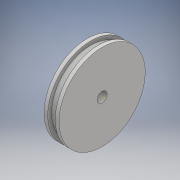
# Autodesk Inventor part: Roue_encodeuse
Saved by Autodesk Inventor 2018 (Build 220112000, 112)
## iProperties
Created: 2019-11-11
Part Number: Roue_encodeuse
Material: Generic
Document SubType Name: Modeling
Designer: hugo
Density: 1 g/cm^3
Appearance: Default
Author: hugo
Autodesk Inventor part; units mm, degrees
ref_plane "YZ Plane" through (0, 0, 0) normal (1, 0, 0) x (0, 1, 0)
ref_plane "XZ Plane" through (0, 0, 0) normal (0, 1, 0) x (-1, 0, 0)
ref_plane "XY Plane" through (0, 0, 0) normal (0, 0, 1) x (1, 0, 0)
sketch "Sketch4" plane through (0, 0, 0) normal (0, 1, 0) x (-1, 0, 0)
  line L0 (0, 0) -> (0, 17.25)
  line L1 (0, 17.25) -> (1.5, 17.25)
  line L2 (1.5, 17.25) -> (1.5, 15.75)
  line L3 (1.5, 15.75) -> (4.5, 15.75)
  line L4 (4.5, 15.75) -> (4.5, 17.25)
  line L5 (4.5, 17.25) -> (6, 17.25)
  line L6 (6, 17.25) -> (6, 0)
  line L7 (6, 0) -> (0, 0)
  dimension "d11" = 6
  dimension "d12" = 15.75
  dimension "d13" = 1.5
  dimension "d14" = 3
  constraints: 16 end point, 6 perpendicular, 2 point on line, 1 collinear, 1 vertical
  measures "d11" distance of L6.end L0.start
  measures "d12" distance between parallel lines of L7 L3
  measures "d13" distance of L1.end L2.end
  measures "d14" distance of L2.end L3.end
revolve "Revolution1" add sketch "Sketch4" angle 360 about axis through (-6, 0, 0) along (1, 0, 0)
sketch "Sketch5" plane through (0, 0, 0) normal (1, 0, 0) x (0, 0, -1)
  circle A0 centre (0, 0) radius 2
  dimension "d16" = 4
  constraints: 1 centre point, 1 coincident
  measures "d16" diameter of A0
extrude "Extrusion3" cut sketch "Sketch5" against normal up to next
equation "\"d12\" = 0.5 * Di"
equation "\"d13\" = -0.25 * Di + 0.25 * De"
equation "\"d14\" = ep"
equation "\"Di\" = 31.5"
equation "\"De\" = 37.5"
equation "\"ep\" = 3"
body "Solid2"
